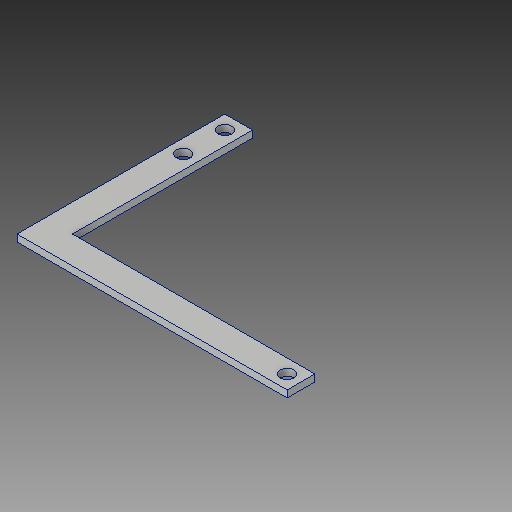
# Autodesk Inventor part: rocker_alt
Saved by Autodesk Inventor 2018.1 (Build 221171000, 171)
## iProperties
Created: 2017-10-26
Part Number: rocker_alt
Material: アルミニウム 6061
Document SubType Name: Modeling
Designer: Kakeru Yamashita
Density: 2.7 g/cm^3
Appearance: アルミニウム - フラット
Mass: 84.5691 g
Surface Area: 164.5 cm^2
Volume: 31.3219 cm^3
Author: Kakeru Yamashita
Autodesk Inventor part; units mm, degrees
ref_plane "YZ Plane" through (0, 0, 0) normal (1, 0, 0) x (0, 1, 0)
ref_plane "XZ Plane" through (0, 0, 0) normal (0, 1, 0) x (-1, 0, 0)
ref_plane "XY Plane" through (0, 0, 0) normal (0, 0, 1) x (1, 0, 0)
sketch "スケッチ1" plane through (0, 0, 0) normal (0, 1, 0) x (-1, 0, 0)
  line L0 (234, 0) -> (-39, 0) projected
  line L1 (0, -180) -> (0, 30) projected
  line L2 (0, 0) -> (195, 0)
  line L3 (195, 0) -> (195, -150)
  line L4 (175, -20) -> (0, -20)
  circle A0 centre (10, -10) radius 5
  circle A1 centre (185, -110) radius 5
  line L5 (195, -150) -> (175, -150)
  circle A2 centre (185, -140) radius 5
  line L6 (175, -20) -> (175, -150)
  dimension "d0" = 195
  dimension "d2" = 20
  dimension "d3" = 150
  dimension "d5" = 10
  dimension "d6" = 10
  dimension "d7" = 10
  dimension "d8" = 10
  dimension "d9" = 10
  dimension "d23" = 40
  dimension "d24" = 10
  dimension "d30" = 10
  dimension "d31" = 10
  dimension "d34" = 20
  constraints: 10 end point, 3 centre point, 2 point on line, 2 vertical, 1 horizontal, 1 perpendicular
  measures "d0" distance of L2.start L2.end
  measures "d2" distance between parallel lines of L2 L4
  measures "d3" distance of L2.end L3.end
  measures "d5" diameter of A0
  measures "d6" distance from line of L1 A0.centre
  measures "d7" distance from line of L0 A0.centre
  measures "d8" diameter of A1
  measures "d9" distance from line of A1.centre L3
  measures "d23" distance from line of L5 A1.centre
  measures "d24" diameter of A2
  measures "d30" distance from line of L5 A2.centre
  measures "d31" distance from line of L3 A2.centre
  measures "d34" distance between parallel lines of L6 L3
extrude "押し出し4" add sketch "スケッチ1" along normal blind 5
